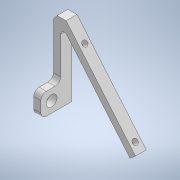
# Autodesk Inventor part: odrive_tester_1
Saved by Autodesk Inventor 2020 (Build 240168000, 168)
## iProperties
Created: 2020-10-15
Part Number: odrive_tester_1
Material: Generic
Document SubType Name: Modeling
Designer: Shuang Peng
Density: 1 g/cm^3
Appearance: Default
Author: Shuang Peng
Autodesk Inventor part; units mm, degrees
ref_plane "YZ Plane" through (0, 0, 0) normal (1, 0, 0) x (0, 1, 0)
ref_plane "XZ Plane" through (0, 0, 0) normal (0, 1, 0) x (-1, 0, 0)
ref_plane "XY Plane" through (0, 0, 0) normal (0, 0, 1) x (1, 0, 0)
sketch "Sketch1" plane through (0, 0, 0) normal (0, 0, 1) x (1, 0, 0)
  line L0 (0, 0) -> (-4, 0)
  line L1 (-4, 0) -> (-4, -40)
  line L2 (-4, -40) -> (0, -40)
  line L3 (0, -40) -> (0, 0)
  line L4 (0, 0) -> (38.5673, -45.9627)
  line L5 (38.5673, -45.9627) -> (41.6314, -43.3915)
  line L6 (41.6314, -43.3915) -> (3.0642, 2.5712)
  line L7 (3.0642, 2.5712) -> (0.493, 5.6353)
  line L8 (0.493, 5.6353) -> (-4, 0)
  dimension "d0" = 4
  dimension "d1" = 40
  dimension "d2" = 60
  dimension "d3" = 4
  dimension "d4" = 60
  dimension "d5" = 4
  dimension "d6" = 40
  constraints: 18 end point, 3 parallel, 2 perpendicular, 1 collinear, 1 horizontal
  measures "d0" distance of L2.end L1.end
  measures "d1" distance of L1.end L0.end
  measures "d2" distance of L0.start L4.end
  measures "d3" distance of L4.end L5.end
  measures "d4" distance of L5.end L6.end
  measures "d5" distance of L6.end L7.end
  measures "d6" angle of L3 L4
extrude "Extrusion1" add sketch "Sketch1" along normal blind 6
fillet "Fillet1" radius 2 1 edges at (0, 0, 3)
sketch "Sketch2" plane through (0.493, 5.6353, 6) normal (0.7660444, 0.6427876, 0) x (0, 0, -1)
  line L0 (6, -64) -> (6, 0) projected
  line L1 (6, 0) -> (0, 0) projected
  line L2 (0, -64) -> (0, 0) projected
  line L3 (6, -64) -> (0, -64) projected
  line L4 (3, -64) -> (3, -59)
  line L5 (3, -59) -> (3, -15.5)
  circle A0 centre (3, -15.5) radius 1.5
  circle A1 centre (3, -59) radius 1.5
  point P0 (6, -4)
  dimension "d10" = 5
  dimension "d11" = 43.5
  dimension "d12" = 3
  dimension "d13" = 3
  constraints: 4 end point, 2 centre point, 2 coincident, 1 midpoint, 1 point on line, 1 vertical
  measures "d10" distance of L4.start L4.end
  measures "d11" distance of L4.end L5.end
  measures "d12" diameter of A0
  measures "d13" diameter of A1
extrude "Extrusion2" cut sketch "Sketch2" against normal blind 6 contours A1 L5 L4 | L4 L5 A1 | A0
sketch "Sketch3" plane through (-4, -40, 0) normal (-1, 0, 0) x (0, 0, 1)
  line L0 (0, 40) -> (0, 0) projected
  line L1 (0, 0) -> (6, 0) projected
  line L2 (6, 40) -> (6, 0) projected
  line L3 (0, 40) -> (6, 40) projected
  line L4 (0, 0) -> (16, 0)
  line L5 (16, 0) -> (16, 10)
  line L6 (16, 10) -> (0, 10)
  line L7 (0, 10) -> (0, 0)
  line L8 (16, 5) -> (11, 5)
  circle A0 centre (11, 5) radius 3
  point P0 (6, 10)
  dimension "d16" = 16
  dimension "d17" = 10
  dimension "d18" = 5
  dimension "d19" = 6
  constraints: 10 end point, 2 horizontal, 2 parallel, 1 centre point, 1 coincident, 1 midpoint, 1 perpendicular
  measures "d16" distance of L6.end L5.end
  measures "d17" distance of L5.end L4.end
  measures "d18" distance of L8.start L8.end
  measures "d19" diameter of A0
extrude "Extrusion3" add sketch "Sketch3" against normal up to surface (4 mm away) contours L6 L5 L4 L2
fillet "Fillet2" radius 3 3 edges at (-2, -30, 6) (-2, -30, 16) (-2, -40, 16)
thicken "Thicken1" operation add thickness 1 both sides no extend neighbours yes toward (0, 1, 0) faces at (-2.6667, -30, 11.6667)
thicken "Thicken2" operation add thickness 1 both sides no extend neighbours yes toward (0, -1, 0) faces at (-2.6667, -40, 4.3333)
thicken "Thicken3" operation add thickness 1 both sides no extend neighbours yes toward (0, 0, 1) faces at (-2.6667, -36, 16)
chamfer "Chamfer1" distance 4 angle 45 1 edges at (0.493, 5.6353, 3)
body "Solid1"
